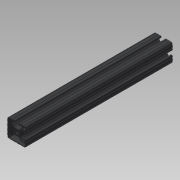
# Autodesk Inventor part: 1502
Saved by Autodesk Inventor 2013 (Build 170138000, 138)
## iProperties
Company: 80/20 Inc.
Created: 2014-04-23
Part Number: 1502
Material: Generic
Document SubType Name: Modeling
Density: 1 g/cm^3
Vendor: 80/20 Inc.
Engineer: Ross Bowman
Designer: Ross Bowman
Catalog Web Link: 8020.net
Material: 6105-T5 Aluminum
Author: Ross Bowman
Keywords: 80/20 , 8020 , T-Slot , Extrusion
Autodesk Inventor part; units mm, degrees
ref_plane "YZ Plane" through (0, 0, 0) normal (1, 0, 0) x (0, 1, 0)
ref_plane "XZ Plane" through (0, 0, 0) normal (0, 1, 0) x (-1, 0, 0)
ref_plane "XY Plane" through (0, 0, 0) normal (0, 0, 1) x (1, 0, 0)
sketch "Sketch1" plane through (0, 0, 0) normal (0, 0, 1) x (1, 0, 0)
  circle A0 centre (0, 0) radius 3.3274
  arc A1 (17.272, 14.478) -> (14.478, 17.272) centre (14.478, 14.478) ccw
  line L0 (17.272, 12.268) -> (17.272, 14.478)
  arc A2 (16.8908, 11.8868) -> (17.272, 12.268) centre (16.8908, 12.268) ccw
  line L1 (12.2428, 11.8868) -> (16.8908, 11.8868)
  arc A3 (11.8616, 12.268) -> (12.2428, 11.8868) centre (12.2428, 12.268) ccw
  line L2 (11.8616, 16.8908) -> (11.8616, 12.268)
  arc A4 (12.2428, 17.272) -> (11.8616, 16.8908) centre (12.2428, 16.8908) ccw
  line L3 (14.478, 17.272) -> (12.2428, 17.272)
  arc A5 (-8.1479, -5.9632) -> (-6.7564, -2.6043) centre (-11.5062, -2.6043) ccw
  line L4 (-11.1176, -8.9324) -> (-8.1479, -5.9632)
  arc A6 (-11.1176, -8.9324) -> (-11.2442, -9.0999) centre (-10.5788, -9.4713) ccw
  line L5 (-12.246, -10.8947) -> (-11.2442, -9.0999)
  arc A7 (-12.3726, -11.0622) -> (-12.246, -10.8947) centre (-12.9114, -10.5234) ccw
  line L6 (-16.6213, -15.3102) -> (-12.3726, -11.0622)
  arc A8 (-17.272, -15.0406) -> (-16.6213, -15.3102) centre (-16.8908, -15.0406) ccw
  line L7 (-17.272, 14.4815) -> (-17.272, -15.0406)
  arc A9 (-14.478, 17.2755) -> (-17.272, 14.4815) centre (-14.478, 14.4815) ccw
  line L8 (-12.4462, 17.2755) -> (-14.478, 17.2755)
  arc A10 (-12.065, 16.8943) -> (-12.4462, 17.2755) centre (-12.4462, 16.8943) ccw
  line L9 (-12.065, 11.195) -> (-12.065, 16.8943)
  arc A11 (-12.065, 11.195) -> (-11.1349, 8.9497) centre (-8.89, 11.195) ccw
  line L10 (-8.1479, 5.9632) -> (-11.1349, 8.9497)
  arc A12 (-6.7564, 2.6043) -> (-8.1479, 5.9632) centre (-11.5062, 2.6043) ccw
  line L11 (-6.7564, -2.6043) -> (-6.7564, 2.6043)
  arc A13 (-9.2978, -11.3824) -> (-9.1308, -11.2561) centre (-9.6695, -10.7172) ccw
  line L12 (-6.0215, -8.1473) -> (-9.1308, -11.2561)
  arc A14 (-2.6631, -6.7564) -> (-6.0215, -8.1473) centre (-2.6631, -11.5062) ccw
  line L13 (2.6631, -6.7564) -> (-2.6631, -6.7564)
  arc A15 (6.0215, -8.1473) -> (2.6631, -6.7564) centre (2.6631, -11.5062) ccw
  line L14 (8.9803, -11.1056) -> (6.0215, -8.1473)
  arc A16 (8.9803, -11.1056) -> (11.2251, -12.0354) centre (11.2251, -8.8604) ccw
  line L15 (16.8908, -12.0354) -> (11.2251, -12.0354)
  arc A17 (17.272, -12.4166) -> (16.8908, -12.0354) centre (16.8908, -12.4166) ccw
  line L16 (17.272, -14.478) -> (17.272, -12.4166)
  arc A18 (14.478, -17.272) -> (17.272, -14.478) centre (14.478, -14.478) ccw
  line L17 (-14.9908, -17.272) -> (14.478, -17.272)
  arc A19 (-15.2603, -16.6212) -> (-14.9908, -17.272) centre (-14.9908, -16.8908) ccw
  line L18 (-11.0116, -12.3733) -> (-15.2603, -16.6212)
  arc A20 (-10.8446, -12.247) -> (-11.0116, -12.3733) centre (-10.4729, -12.9121) ccw
  line L19 (-9.2978, -11.3824) -> (-10.8446, -12.247)
  line L20 (15.879, -6.7506) -> (15.879, -8.9192)
  arc A21 (14.609, -10.1892) -> (15.879, -8.9192) centre (14.609, -8.9192) ccw
  line L21 (14.609, -10.1892) -> (12.7428, -10.1892)
  arc A22 (12.1142, -9.9289) -> (12.7428, -10.1892) centre (12.7428, -9.3002) ccw
  line L22 (12.1142, -9.9289) -> (8.1479, -5.9632)
  arc A23 (6.7564, -2.6043) -> (8.1479, -5.9632) centre (11.5062, -2.6043) ccw
  line L23 (6.7564, -2.6043) -> (6.7564, 2.6043)
  arc A24 (8.1479, 5.9632) -> (6.7564, 2.6043) centre (11.5062, 2.6043) ccw
  line L24 (8.1479, 5.9632) -> (12.1142, 9.9289)
  arc A25 (12.7428, 10.1892) -> (12.1142, 9.9289) centre (12.7428, 9.3002) ccw
  line L25 (12.7428, 10.1892) -> (14.609, 10.1892)
  arc A26 (15.879, 8.9192) -> (14.609, 10.1892) centre (14.609, 8.9192) ccw
  line L26 (15.879, 8.9192) -> (15.879, 6.7506)
  line L27 (15.879, 6.7506) -> (14.986, 6.7506)
  line L28 (14.986, 6.7506) -> (14.986, 5.5753)
  arc A27 (14.986, 5.5753) -> (16.5608, 4.0005) centre (16.5608, 5.5753) ccw
  line L29 (16.5608, 4.0005) -> (17.4752, 4.0005)
  arc A28 (17.4752, 4.0005) -> (19.05, 5.5753) centre (17.4752, 5.5753) ccw
  line L30 (19.05, 5.5753) -> (19.05, 7.9756)
  arc A29 (19.05, 9.4996) -> (19.05, 7.9756) centre (19.05, 8.7376) ccw
  line L31 (19.05, 9.4996) -> (19.05, 14.3256)
  arc A30 (19.05, 15.8496) -> (19.05, 14.3256) centre (19.05, 15.0876) ccw
  line L32 (19.05, 15.8496) -> (19.05, 15.875)
  arc A31 (19.05, 15.875) -> (15.875, 19.05) centre (15.875, 15.875) ccw
  line L33 (15.875, 19.05) -> (15.8496, 19.05)
  arc A32 (14.3256, 19.05) -> (15.8496, 19.05) centre (15.0876, 19.05) ccw
  line L34 (14.3256, 19.05) -> (9.4996, 19.05)
  arc A33 (7.9756, 19.05) -> (9.4996, 19.05) centre (8.7376, 19.05) ccw
  line L35 (7.9756, 19.05) -> (5.6388, 19.05)
  arc A34 (5.6388, 19.05) -> (4.064, 17.4752) centre (5.6388, 17.4752) ccw
  line L36 (4.064, 17.4752) -> (4.064, 16.5608)
  arc A35 (4.064, 16.5608) -> (5.6388, 14.986) centre (5.6388, 16.5608) ccw
  line L37 (5.6388, 14.986) -> (6.8141, 14.986)
  line L38 (6.8141, 14.986) -> (6.8141, 15.8247)
  line L39 (6.8141, 15.8247) -> (9.017, 15.8247)
  arc A36 (10.287, 14.5547) -> (9.017, 15.8247) centre (9.017, 14.5547) ccw
  line L40 (10.287, 14.5547) -> (10.287, 12.7802)
  arc A37 (10.0267, 12.1519) -> (10.287, 12.7802) centre (9.3985, 12.7802) ccw
  line L41 (10.0267, 12.1519) -> (6.0215, 8.1473)
  arc A38 (2.6631, 6.7564) -> (6.0215, 8.1473) centre (2.6631, 11.5062) ccw
  line L42 (2.6631, 6.7564) -> (-2.6631, 6.7564)
  arc A39 (-6.0215, 8.1473) -> (-2.6631, 6.7564) centre (-2.6631, 11.5062) ccw
  line L43 (-6.0215, 8.1473) -> (-10.0267, 12.1519)
  arc A40 (-10.287, 12.7802) -> (-10.0267, 12.1519) centre (-9.3985, 12.7802) ccw
  line L44 (-10.287, 12.7802) -> (-10.287, 14.5547)
  arc A41 (-9.017, 15.8247) -> (-10.287, 14.5547) centre (-9.017, 14.5547) ccw
  line L45 (-9.017, 15.8247) -> (-6.8141, 15.8247)
  line L46 (-6.8141, 15.8247) -> (-6.8141, 14.986)
  line L47 (-6.8141, 14.986) -> (-5.6388, 14.986)
  arc A42 (-5.6388, 14.986) -> (-4.064, 16.5608) centre (-5.6388, 16.5608) ccw
  line L48 (-4.064, 16.5608) -> (-4.064, 17.4752)
  arc A43 (-4.064, 17.4752) -> (-5.6388, 19.05) centre (-5.6388, 17.4752) ccw
  line L49 (-5.6388, 19.05) -> (-7.9756, 19.05)
  arc A44 (-9.4996, 19.05) -> (-7.9756, 19.05) centre (-8.7376, 19.05) ccw
  line L50 (-9.4996, 19.05) -> (-14.3256, 19.05)
  arc A45 (-15.8496, 19.05) -> (-14.3256, 19.05) centre (-15.0876, 19.05) ccw
  line L51 (-15.8496, 19.05) -> (-15.875, 19.05)
  arc A46 (-15.875, 19.05) -> (-19.05, 15.875) centre (-15.875, 15.875) ccw
  line L52 (-19.05, 15.875) -> (-19.05, 15.8496)
  arc A47 (-19.05, 14.3256) -> (-19.05, 15.8496) centre (-19.05, 15.0876) ccw
  line L53 (-19.05, 14.3256) -> (-19.05, 9.4996)
  arc A48 (-19.05, 7.9756) -> (-19.05, 9.4996) centre (-19.05, 8.7376) ccw
  line L54 (-19.05, 7.9756) -> (-19.05, 0.762)
  arc A49 (-19.05, -0.762) -> (-19.05, 0.762) centre (-19.05, 0) ccw
  line L55 (-19.05, -0.762) -> (-19.05, -7.9756)
  arc A50 (-19.05, -9.4996) -> (-19.05, -7.9756) centre (-19.05, -8.7376) ccw
  line L56 (-19.05, -9.4996) -> (-19.05, -14.3256)
  arc A51 (-19.05, -15.8496) -> (-19.05, -14.3256) centre (-19.05, -15.0876) ccw
  line L57 (-19.05, -15.8496) -> (-19.05, -15.875)
  arc A52 (-19.05, -15.875) -> (-15.875, -19.05) centre (-15.875, -15.875) ccw
  line L58 (-15.875, -19.05) -> (-15.8496, -19.05)
  arc A53 (-14.3256, -19.05) -> (-15.8496, -19.05) centre (-15.0876, -19.05) ccw
  line L59 (-14.3256, -19.05) -> (-9.4996, -19.05)
  arc A54 (-7.9756, -19.05) -> (-9.4996, -19.05) centre (-8.7376, -19.05) ccw
  line L60 (-7.9756, -19.05) -> (-0.762, -19.05)
  arc A55 (0.762, -19.05) -> (-0.762, -19.05) centre (0, -19.05) ccw
  line L61 (0.762, -19.05) -> (7.9756, -19.05)
  arc A56 (9.4996, -19.05) -> (7.9756, -19.05) centre (8.7376, -19.05) ccw
  line L62 (9.4996, -19.05) -> (14.3256, -19.05)
  arc A57 (15.8496, -19.05) -> (14.3256, -19.05) centre (15.0876, -19.05) ccw
  line L63 (15.8496, -19.05) -> (15.875, -19.05)
  arc A58 (15.875, -19.05) -> (19.05, -15.875) centre (15.875, -15.875) ccw
  line L64 (19.05, -15.875) -> (19.05, -15.8496)
  arc A59 (19.05, -14.3256) -> (19.05, -15.8496) centre (19.05, -15.0876) ccw
  line L65 (19.05, -14.3256) -> (19.05, -9.4996)
  arc A60 (19.05, -7.9756) -> (19.05, -9.4996) centre (19.05, -8.7376) ccw
  line L66 (19.05, -7.9756) -> (19.05, -5.5753)
  arc A61 (19.05, -5.5753) -> (17.4752, -4.0005) centre (17.4752, -5.5753) ccw
  line L67 (17.4752, -4.0005) -> (16.5608, -4.0005)
  arc A62 (16.5608, -4.0005) -> (14.986, -5.5753) centre (16.5608, -5.5753) ccw
  line L68 (14.986, -5.5753) -> (14.986, -6.7506)
  line L69 (14.986, -6.7506) -> (15.879, -6.7506)
  constraints: 140 end point, 124 point on circle, 63 centre point
extrude "Extrusion1" add sketch "Sketch1" against normal blind 304.8
body "Solid1"
